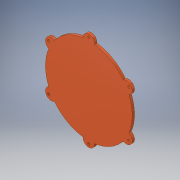
# Autodesk Inventor part: base_plate
Saved by Autodesk Inventor 2017 (Build 210142000, 142)
## iProperties
Created: 2017-01-13
Part Number: base_plate
Material: Phenolic Resin
Document SubType Name: Modeling
Designer: Canton
Density: 1.38 g/cm^3
Appearance: Smooth - Light Orange
Author: Canton
Autodesk Inventor part; units mm, degrees
ref_plane "YZ Plane" through (0, 0, 0) normal (1, 0, 0) x (0, 1, 0)
ref_plane "XZ Plane" through (0, 0, 0) normal (0, 1, 0) x (-1, 0, 0)
ref_plane "XY Plane" through (0, 0, 0) normal (0, 0, 1) x (1, 0, 0)
sketch "Sketch2" plane through (0, 0, 0) normal (0, 0, 1) x (1, 0, 0)
  arc A0 (7.4831, 55.3969) -> (-7.4831, 55.3969) centre (0, 55.9) ccw
  circle A1 centre (0, 59.65) radius 1.5
  arc A2 (-44.2335, 34.179) -> (-51.7166, 21.2179) centre (-48.4108, 27.95) ccw
  circle A3 centre (-51.6584, 29.825) radius 1.5
  arc A4 (-51.7166, -21.2179) -> (-44.2335, -34.179) centre (-48.4108, -27.95) ccw
  circle A5 centre (-51.6584, -29.825) radius 1.5
  arc A6 (-7.4831, -55.3969) -> (7.4831, -55.3969) centre (0, -55.9) ccw
  circle A7 centre (0, -59.65) radius 1.5
  arc A8 (44.2335, -34.179) -> (51.7166, -21.2179) centre (48.4108, -27.95) ccw
  circle A9 centre (51.6584, -29.825) radius 1.5
  arc A10 (51.7166, 21.2179) -> (44.2335, 34.179) centre (48.4108, 27.95) ccw
  circle A11 centre (51.6584, 29.825) radius 1.5
  arc A12 (-7.4831, 55.3969) -> (-44.2335, 34.179) centre (0, 0) ccw
  arc A13 (-51.7166, 21.2179) -> (-51.7166, -21.2179) centre (0, 0) ccw
  arc A14 (-44.2335, -34.179) -> (-7.4831, -55.3969) centre (0, 0) ccw
  arc A15 (7.4831, -55.3969) -> (44.2335, -34.179) centre (0, 0) ccw
  arc A16 (51.7166, -21.2179) -> (51.7166, 21.2179) centre (0, 0) ccw
  arc A17 (44.2335, 34.179) -> (7.4831, 55.3969) centre (0, 0) ccw
  dimension "d12" = 3
  dimension "d15" = 360
  dimension "d20" = 55.9
  constraints: 24 point on circle, 18 centre point, 1 coincident, 37 other
  measures "d12" diameter of A1
  measures "d20" radius of A13
extrude "Extrusion1" add sketch "Sketch2" along normal blind 3
body "Solid1"
